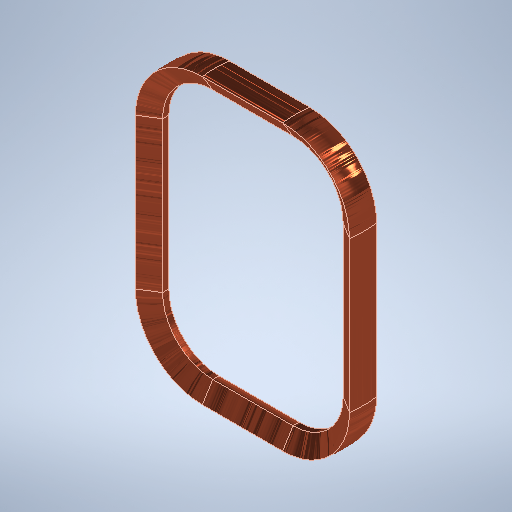
# Autodesk Inventor part: single_coil
Saved by Autodesk Inventor 2025 (Build 290162000, 162)
## iProperties
Created: 2026-08-14
Part Number: single_coil
Material: Ogólny
Document SubType Name: Modeling
Designer: zzapa
Density: 1 g/cm^3
Appearance: Przewód nawojowy
Author: zzapa
Autodesk Inventor part; units mm, degrees
ref_plane "YZ Plane" through (0, 0, 0) normal (1, 0, 0) x (0, 1, 0)
ref_plane "XZ Plane" through (0, 0, 0) normal (0, 1, 0) x (-1, 0, 0)
ref_plane "XY Plane" through (0, 0, 0) normal (0, 0, 1) x (1, 0, 0)
sketch "Szkic1" plane through (0, 0, 0) normal (0, 1, 0) x (-1, 0, 0)
  line L0 (30.1, 0) -> (-30.1, 0) projected
  circle A0 centre (0, 0) radius 18
  circle A1 centre (0, 0) radius 21.5
  line L1 (17.9892, -0.6225) -> (21.3298, -2.7)
  line L2 (17.9892, 0.6225) -> (21.3298, 2.7)
  point P0 (21.3298, 2.7)
  point P1 (17.9892, 0.6225)
  dimension "d4" = 43
  dimension "d5" = 36
  dimension "d6" = 5.4
  dimension "d7" = 1.245
  constraints: 4 end point, 2 coincident, 2 symmetric about line, 6 other
  measures "d6" distance of L1.end L2.end
  measures "d7" distance of L1.start L2.start
sketch3d "Szkic 3D2"
  line L0 (18, 15, 0) -> (18, -15, 0)
  arc A0 (18, -15, 0) -> (8, -25, 0) centre (8, -15, 0) ccw
  line L1 (8, -25, 0) -> (-8, -25, 0)
  arc A1 (-8, -25, 0) -> (-18, -15, 0) centre (-8, -15, 0) ccw
  line L2 (-18, -15, 0) -> (-18, 15, 0)
  arc A2 (-18, 15, 0) -> (-8, 25, 0) centre (-8, 15, 0) ccw
  line L3 (-8, 25, 0) -> (8, 25, 0)
  arc A3 (8, 25, 0) -> (18, 15, 0) centre (8, 15, 0) ccw
  dimension "d9" = 50
  dimension "d10" = 36
  dimension "d11" = 10
  dimension "d12" = 10
  dimension "d13" = 10
  dimension "d14" = 10
sweep "Przeciągnięcie2" add profiles "Szkic1" path "Szkic 3D2" picked at (20.2478, -1.7084) picked at (20.2478, 1.7084) contours A1 L1 A0 L0 | L0 A0 L2 A1
equation "\"d12\" = d11"
equation "\"d13\" = d11"
equation "\"d14\" = d11"
